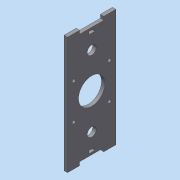
# Autodesk Inventor part: Front-Inner
Saved by Autodesk Inventor 2016 SP1 (Build 200210100, 210)
## iProperties
Created: 2016-03-01
Part Number: Front-Inner
Material: Generic
Document SubType Name: Modeling
Designer: Mohamed A.
Density: 1 g/cm^3
Appearance: Default
Author: Mohamed A.
Autodesk Inventor part; units mm, degrees
ref_plane "YZ Plane" through (0, 0, 0) normal (1, 0, 0) x (0, 1, 0)
ref_plane "XZ Plane" through (0, 0, 0) normal (0, 1, 0) x (-1, 0, 0)
ref_plane "XY Plane" through (0, 0, 0) normal (0, 0, 1) x (1, 0, 0)
sketch "Sketch2" plane through (0, 0, 0) normal (1, 0, 0) x (0, 1, 0)
  circle A0 centre (0, 0) radius 11.5
  line L0 (-29.4, 0) -> (29.4, 0) construction
  line L1 (0, -71.4) -> (0, 71.4) construction
  line L2 (21, 51) -> (10.5, 51)
  line L3 (-21, 51) -> (-21, -51)
  line L4 (-21, -51) -> (-10.5, -51)
  line L5 (21, -51) -> (21, 51)
  line L6 (21, -21) -> (-21, -21) construction
  line L7 (21, 21) -> (-21, 21) construction
  circle A1 centre (15.5, 15.5) radius 1.4
  circle A2 centre (-15.5, 15.5) radius 1.4
  circle A3 centre (-15.5, -15.5) radius 1.4
  circle A4 centre (15.5, -15.5) radius 1.4
  circle A5 centre (0, -30.8333) radius 3.9
  circle A6 centre (0, 30.8333) radius 3.9
  line L8 (21, -48) -> (10.5, -48)
  line L9 (10.5, -51) -> (10.5, -48)
  line L10 (-10.5, -48) -> (-10.5, -51)
  line L11 (10.5, -48) -> (-10.5, -48)
  line L12 (-10.5, -48) -> (-21, -48)
  line L13 (-10.5, -51) -> (10.5, -51)
  line L14 (10.5, -51) -> (21, -51)
  line L15 (21, 48) -> (10.5, 48)
  line L16 (10.5, 51) -> (10.5, 48)
  line L17 (-10.5, 48) -> (-10.5, 51)
  line L18 (10.5, 48) -> (-10.5, 48)
  line L19 (-10.5, 48) -> (-21, 48)
  line L20 (10.5, 51) -> (-10.5, 51)
  line L21 (-10.5, 51) -> (-21, 51)
  line L22 (2.65, -43.6) -> (-2.65, -43.6)
  line L23 (-2.65, -43.6) -> (-2.65, -46)
  line L24 (-2.65, -46) -> (2.65, -46)
  line L25 (2.65, -46) -> (2.65, -43.6)
  line L26 (2.65, 43.6) -> (-2.65, 43.6)
  line L27 (-2.65, 43.6) -> (-2.65, 46)
  line L28 (-2.65, 46) -> (2.65, 46)
  line L29 (2.65, 46) -> (2.65, 43.6)
  dimension "d0" = 23
  dimension "d1" = 42
  dimension "d2" = 102
  dimension "d4" = 2.8
  dimension "d5" = 5.5
  dimension "d6" = 5.5
  dimension "d9" = 360
  dimension "d11" = 7.8
  dimension "d13" = 7.8
  dimension "d15" = 3
  dimension "d16" = 21
  dimension "d17" = 5.3
  dimension "d18" = 2.4
  dimension "d19" = 5
  dimension "d25" = 30.8333
  dimension "d26" = 30.8333
  constraints: 56 end point, 14 perpendicular, 12 parallel, 11 point on line, 10 symmetric about line, 7 centre point, 5 horizontal, 1 coincident, 1 midpoint, 14 other
  measures "d0" diameter of A0
  measures "d1" distance of L5.start L3.end
  measures "d2" distance of L3.end L3.start
  measures "d4" diameter of A1
  measures "d5" distance from line of A1.centre L5
  measures "d6" distance from line of L7 A1.centre
  measures "d11" diameter of A5
  measures "d13" diameter of A6
  measures "d15" distance between parallel lines of L4 L8
  measures "d16" distance between parallel lines of L10 L9
  measures "d17" distance of L24.end L23.end
  measures "d18" distance of L23.end L22.end
  measures "d19" distance between parallel lines of L13 L24
  measures "d25" distance of point (0, 0) A5.centre
  measures "d26" distance of point (0, 0) A6.centre
extrude "Extrusion1" add sketch "Sketch2" along normal blind 3 contours L5 L15 L16 L2 | L5 L8 L11 L12 L3 L19 L18 L15 | L17 L19 L3 L21 | L5 L14 L9 L8 | L10 L4 L3 L12
equation "\"d16\" = 0.5 * d1"
body "Solid1"
